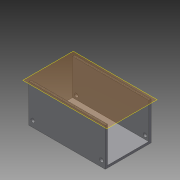
# Autodesk Inventor part: EE_Base-SquareBar-Rev3
Saved by Autodesk Inventor 2015 (Build 190159000, 159)
## iProperties
Created: 2017-01-10
Part Number: EE_Base-SquareBar-Rev3
Material: Generic
Document SubType Name: Modeling
Designer: Guy
Density: 1 g/cm^3
Appearance: Default
Author: Guy
Autodesk Inventor part; units mm, degrees
ref_plane "YZ Plane" through (0, 0, 0) normal (1, 0, 0) x (0, 1, 0)
ref_plane "XZ Plane" through (0, 0, 0) normal (0, 1, 0) x (-1, 0, 0)
ref_plane "XY Plane" through (0, 0, 0) normal (0, 0, 1) x (1, 0, 0)
sketch "Sketch6" plane through (0, 0, 0) normal (0, 0, 1) x (1, 0, 0)
  line L0 (0, 0) -> (100, 0)
  line L1 (100, 0) -> (100, 60)
  line L2 (100, 60) -> (0, 60)
  line L3 (0, 60) -> (0, 0)
  dimension "d18" = 60
  dimension "d19" = 100
  constraints: 8 end point, 2 parallel, 1 horizontal, 1 perpendicular
  measures "d18" distance between parallel lines of L0 L2
  measures "d19" distance of L1.end L2.end
extrude "Extrusion4" add sketch "Sketch6" along normal blind 100
sketch "Sketch7" plane through (100, 0, 0) normal (1, 0, 0) x (0, 0, -1)
  line L0 (0, 0) -> (0, 60) projected
  line L1 (0, 60) -> (-100, 60) projected
  line L2 (-100, 0) -> (-100, 60) projected
  line L3 (0, 0) -> (-100, 0) projected
  line L4 (-97, 3) -> (-3, 3)
  line L5 (-3, 3) -> (-3, 57)
  line L6 (-3, 57) -> (-97, 57)
  line L7 (-97, 57) -> (-97, 3)
  point P0 (0, 0)
  dimension "d22" = 3
  dimension "d23" = 3
  dimension "d24" = 3
  dimension "d25" = 3
  constraints: 8 end point, 2 parallel, 1 horizontal, 1 perpendicular
  measures "d22" distance between parallel lines of L1 L6
  measures "d23" distance between parallel lines of L2 L7
  measures "d24" distance between parallel lines of L3 L4
  measures "d25" distance between parallel lines of L0 L5
extrude "Extrusion5" cut sketch "Sketch7" against normal up to next contours L7 L6 L5 L4
sketch "Sketch8" plane through (0, 0, 0) normal (0, -1, 0) x (1, 0, 0)
  line L0 (0, 0) -> (100, 0) projected
  line L1 (100, 0) -> (100, 100) projected
  line L2 (0, 100) -> (100, 100) projected
  line L3 (0, 0) -> (0, 100) projected
  line L4 (100, 3) -> (0, 3) projected
  circle A0 centre (5, 8) radius 2.5
  circle A1 centre (95, 8) radius 2.5
  dimension "d28" = 5
  dimension "d29" = 5
  dimension "d30" = 5
  dimension "d31" = 5
  dimension "d32" = 5
  dimension "d33" = 5
  constraints: 2 centre point
  measures "d28" diameter of A1
  measures "d29" diameter of A0
  measures "d30" distance from line of L4 A0.centre
  measures "d31" distance from line of L3 A0.centre
  measures "d32" distance from line of L1 A1.centre
  measures "d33" distance from line of L4 A1.centre
extrude "Extrusion6" cut sketch "Sketch8" against normal blind 100 contours A0 | A1
sketch "Sketch9" plane through (0, 0, 100) normal (0, 0, 1) x (1, 0, 0)
  line L0 (0, 0) -> (100, 0) projected
  line L1 (100, 0) -> (100, 60) projected
  line L2 (100, 60) -> (0, 60) projected
  line L3 (0, 60) -> (0, 0) projected
  line L4 (100, 57) -> (0, 57) projected
  line L5 (100, 3) -> (0, 3) projected
  circle A0 centre (10, 30) radius 2.5
  dimension "d36" = 5
  dimension "d37" = 30
  dimension "d38" = 10
  constraints: 1 centre point
  measures "d36" diameter of A0
  measures "d37" distance from line of L0 A0.centre
  measures "d38" distance from line of A0.centre L3
extrude "Extrusion7" cut sketch "Sketch9" against normal through all contours A0
ref_plane "Work Plane1" through (0, 0, 50) normal (0, 0, 1) x (1, 0, 0)
body "Solid2"
